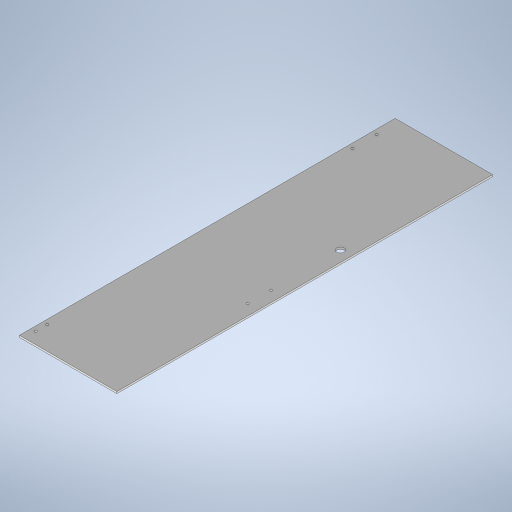
# Autodesk Inventor part: Дверь
Saved by Autodesk Inventor 2023 (Build 270158000, 158)
## iProperties
Created: 2022-04-27
Part Number: Дверь
Material: Типовые
Document SubType Name: Modeling
Designer: User
Density: 1 g/cm^3
Appearance: По умолчанию
Author: User
Autodesk Inventor part; units mm, degrees
ref_plane "YZ Plane" through (0, 0, 0) normal (1, 0, 0) x (0, 1, 0)
ref_plane "XZ Plane" through (0, 0, 0) normal (0, 1, 0) x (-1, 0, 0)
ref_plane "XY Plane" through (0, 0, 0) normal (0, 0, 1) x (1, 0, 0)
sketch "Эскиз1" plane through (0, 0, 0) normal (0, 1, 0) x (-1, 0, 0)
  line L0 (0, 0) -> (-210, 0)
  line L1 (-210, 0) -> (-210, -810)
  line L2 (-210, -810) -> (0, -810)
  line L3 (0, -810) -> (0, 0)
  line L4 (-186.9152, -405) -> (-186.9152, -395)
  line L5 (-186.9152, -395) -> (-186.9152, -305)
  line L6 (-186.9152, -305) -> (-186.9152, -505)
  circle A0 centre (-186.9152, -505) radius 8
  circle A1 centre (-186.9152, -305) radius 2.5
  line L7 (-186.9152, -305) -> (-186.9152, -310)
  line L8 (-186.9152, -310) -> (-186.9152, -355)
  circle A2 centre (-186.9152, -355) radius 2.5
  line L9 (0, 0) -> (0, -50)
  line L10 (0, -50) -> (-10, -50)
  line L11 (0, -810) -> (0, -760)
  line L12 (0, -760) -> (-10, -760)
  circle A3 centre (-10, -760) radius 2.5
  circle A4 centre (-10, -707.8561) radius 2.5
  circle A5 centre (-10, -50) radius 2.5
  circle A6 centre (-10, -25) radius 2.5
  dimension "d0" = 210
  dimension "d1" = 810
  dimension "d2" = 10
  dimension "d3" = 90
  dimension "d4" = 200
  dimension "d5" = 16
  dimension "d6" = 5
  dimension "d7" = 5
  dimension "d8" = 45
  dimension "d9" = 5
  dimension "d10" = 50
  dimension "d11" = 10
  dimension "d12" = 50
  dimension "d13" = 10
  dimension "d14" = 5
  dimension "d15" = 5
  dimension "d16" = 5
  dimension "d17" = 5
  constraints: 26 end point, 7 centre point, 6 point on line, 5 coincident, 3 perpendicular, 2 parallel, 1 horizontal
  measures "d0" distance of L2.end L1.end
  measures "d1" distance of L1.end L0.end
  measures "d2" distance of L4.start L4.end
  measures "d3" distance of L4.end L5.end
  measures "d4" distance of L5.end L6.end
  measures "d5" diameter of A0
  measures "d6" diameter of A1
  measures "d7" distance of L7.start L7.end
  measures "d8" distance of L7.end L8.end
  measures "d9" diameter of A2
  measures "d10" distance of L0.start L9.end
  measures "d11" distance of L9.end L10.end
  measures "d12" distance of L2.end L11.end
  measures "d13" distance of L11.end L12.end
  measures "d14" diameter of A3
  measures "d15" diameter of A4
  measures "d16" diameter of A5
  measures "d17" diameter of A6
extrude "Выдавливание1" add sketch "Эскиз1" along normal blind 4
